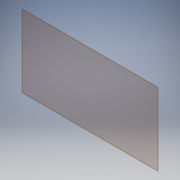
# Autodesk Inventor part: Intake_backboard
Saved by Autodesk Inventor 2018 (Build 220112000, 112)
## iProperties
Created: 2018-09-10
Part Number: Intake_backboard
Material: Generic
Document SubType Name: Modeling
Designer: baoan
Density: 1 g/cm^3
Appearance: Polycarbonate - Smoked
Author: baoan
Autodesk Inventor part; units mm, degrees
ref_plane "YZ Plane" through (0, 0, 0) normal (1, 0, 0) x (0, 1, 0)
ref_plane "XZ Plane" through (0, 0, 0) normal (0, 1, 0) x (-1, 0, 0)
ref_plane "XY Plane" through (0, 0, 0) normal (0, 0, 1) x (1, 0, 0)
sketch "Sketch1" plane through (0, 0, 0) normal (0, 0, 1) x (1, 0, 0)
  line L0 (279.4, -149.225) -> (-279.4, -149.225)
  line L1 (-279.4, -149.225) -> (-279.4, 149.225)
  line L2 (-279.4, 149.225) -> (279.4, 149.225)
  line L3 (279.4, 149.225) -> (279.4, -149.225)
  line L4 (279.4, -149.225) -> (-279.4, 149.225) construction
  line L5 (-279.4, -149.225) -> (279.4, 149.225) construction
  point P0 (0, 0)
  dimension "d0" = 558.8
  dimension "d1" = 298.45
  constraints: 12 end point, 2 midpoint, 2 parallel, 1 horizontal, 1 perpendicular
  measures "d0" distance of L1.end L2.end
  measures "d1" distance of L0.end L1.end
extrude "Extrusion1" add sketch "Sketch1" along normal mid plane 3.175
body "Solid1"
